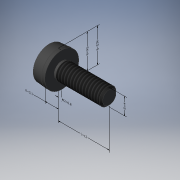
# Autodesk Inventor part: ART 48240 - DIN 6900-1 Z0 T M4x12.0 mm - A2
Saved by Autodesk Inventor 2019 (Build 230136000, 136)
## iProperties
Created: 2022-09-09
Part Number: ART 48240 - DIN 6900-1 Z0 T M4x12.0 mm - A2
Material: Generic
Catalog Web Link: www.cadenas.de
Description: DIN 6900-1 Z0 T stainless steel A2 plain-Torx SEMS screws with small flat washer
Vendor: ART
Document SubType Name: Modeling
Designer: psAdmin
Manufacturer: ART
Mass: 0.285727 g
Surface Area: 3.33062 cm^2
Volume: 0.285727 cm^3
Density: 1 g/cm^3
Appearance: PSOLRGB-192-192-192
Category: PARTsolutions
Company: ART
Title: A.R.T. 48240 - DIN 6900-1 Z0 T M4x12.0 mm - A2
Author: Cadenas PARTsolutions
Comments: Torx SEMS screws with small flat washer
PSOL_IDENT_0: {$CADENAS_DATA/23d-libs/art/mz/kombischrauben/din_6900_1_z1_z0_t/din_6900_1_z0_t_a2.prj},264 {VTYP=3
PSOL_IDENT_1: D},{NB=ART 48240 - DIN 6900-1 Z0 T M4x12.0 mm - A2},{LINA=A.R.T. 48240 - DIN 6900-1 Z0 T M4x12.0 mm
PSOL_IDENT_2: - A2},{NN=DIN 6900-1 Z0 T stainless steel A2 plain},{DATE=17.05.2021 04:49:58},{GEOMDATE=29.04.2021
PSOL_IDENT_3: 06:09:35},{VERSION=},{LINEID=260},{WBVAR=},{WBNUMERIC=}  {NB=ART 48240 - DIN 6900-1 Z0 T M4x12.0 mm
PSOL_IDENT_4: - A2},{LINA=A.R.T. 48240 - DIN 6900-1 Z0 T M4x12.0 mm - A2},{KT=X},{IDNR=},{NENN=M4x12.0 mm - A2},{A
PSOL_IDENT_5: RTNR=48240},{TYP=DIN 6900-1 Z0 T},{ZTN=7318 1595},{MT=Metall},{MAT=Edelstahl},{GUETE=A2},{OBERFLAECH
PSOL_IDENT_6: E=blank},{DINSCHRAUBE=DIN 7985 - Torx},{DINSCHEIBE=DIN 6902C - Unterlegscheibe ähnl. DIN 433 (Z0)},{
PSOL_IDENT_7: ISO=ISO 10644 S11-S},{D=4.0},{D3=3.141},{P=0.700},{L=12},{A=1.400},{B=10.6},{BX=22},{DK=8},{AD2=8.0}
PSOL_IDENT_8: ,{K=3.1},{H2=0.8},{ANTRIEB=Torx T20},{ANTRIEB1=Torx},{A1=3.950},{T=1.660},{DA=4.700},{R=0.200},{RF=8
PSOL_IDENT_9: .000},{V=2.000},{X=1.750},{DIN962FTHREAD=0},{VERS=1},{DIST=0.8},{CNSAVOID=0},{CNSNN=DIN 7985},{CNSOR
PSOL_IDENT_10: DER=DIN 7985 M4x12.0 mm - A2},{LINK1=www.artgmbh.com},{LWS=https://www.artgmbh.com/montagezubehoer-k
PSOL_IDENT_11: ombischrauben/kombischrauben/din-6900-1-z1-kombischrauben-torx-mit-unterlegscheibe/},{LINK2=https://
PSOL_IDENT_12: www.artgmbh.com/media/static/pdf/ART_ELEKTROMECHANIK_Gesamtkatalog.pdf},{LKS=https://www.artgmbh.com
PSOL_IDENT_13: /media/static/pdf/ART_ELEKTROMECHANIK_Gesamtkatalog.pdf}
NB: ART 48240 - DIN 6900-1 Z0 T M4x12.0 mm - A2
NN: DIN 6900-1 Z0 T stainless steel A2 plain
NT: Torx SEMS screws with small flat washer
NBSYN: ART $ARTNR. - $TYP. $NENN.
LINA: A.R.T. 48240 - DIN 6900-1 Z0 T M4x12.0 mm - A2
CATALOG: A.R.T. Elektromechanik
ROWDESC: M4x12.0 mm - A2
OFFICIAL_STANDARD_NUMBERS: DIN 6900
ARTNR: 48240
TYP: DIN 6900-1 Z0 T
ZTN: 7318 1595
MT: Metal
MAT: stainless steel
GUETE: A2
OBERFLAECHE: plain
DINSCHRAUBE: DIN 7985 - Torx
DINSCHEIBE: DIN 6902C - Flat washer similar to DIN 433 (Z0)
ISO: ISO 10644 S11-S
D: 4
P: 0.7
L: 12
DK: 8
AD2: 8
K: 3.1
H2: 0.8
ANTRIEB: Torx T20
LINK1: www.artgmbh.com
LINK2: https://www.artgmbh.com/media/static/pdf/ART_ELEKTROMECHANIK_Gesamtkatalog.pdf
SUPPLIER: ART
ARTICLENO: ART 48240 - DIN 6900-1 Z0 T M4x12.0 mm - A2
BOMINFO: A.R.T. 48240 - DIN 6900-1 Z0 T M4x12.0 mm - A2
CREATOR: CADENAS GmbH
Autodesk Inventor part; units mm, degrees
sketch "Skizze_3" plane through (0, 0, 0) normal (0, 0, 1) x (1, 0, 0)
  line L0 (12, 0) -> (-3.1, 0)
  line L1 (-3.1, 0) -> (-3.1, 4)
  line L2 (-3.1, 4) -> (0, 4)
  line L3 (0, 4) -> (0, 2)
  line L4 (0, 2) -> (11.5705, 2)
  line L5 (11.5705, 2) -> (12, 1.5705)
  line L6 (12, 1.5705) -> (12, 0)
  line L7 (12, 0) -> (-3.1, 0)
  constraints: 16 end point
revolve "Revolution1" add sketch "Skizze_3" angle 360 about axis through (12, 0, 0) along (1, 0, 0)
thread "Thread1" size "M4x0.7" class "6g" standard "ISO Metric profile" length 10.1705
sketch "Sketch_6" plane through (0, 0, 0) normal (0, 0, 1) x (1, 0, 0)
  line L0 (1.4, 0) -> (0, 0)
  line L1 (0, 2.6111) -> (0, 2.35)
  arc A0 (0, 2.35) -> (0.0908, 2.1825) centre (0.2, 2.35) ccw
  line L2 (0.0908, 2.1825) -> (0.7, 1.7853)
  line L3 (0.7, 1.7853) -> (1.4, 2)
  line L4 (1.4, 2) -> (1.4, 2.6111)
  line L5 (1.4, 2.6111) -> (0, 2.6111)
  constraints: 12 end point, 2 point on circle, 1 centre point
revolve "Revolution2" cut sketch "Sketch_6" angle 360 about axis through (1.4, 0, 0) along (1, 0, 0)
sketch "Sketch_2" plane through (0, 0, 0) normal (0, 0, 1) x (1, 0, 0)
  line L0 (0.7, 0) -> (-0.2, 0)
  line L1 (-0.2, 2.6111) -> (-0.2, 1.5705)
  line L2 (-0.2, 1.5705) -> (0.7, 1.5705)
  line L3 (0.7, 1.5705) -> (0.7, 1.7853)
  line L4 (0.7, 1.7853) -> (0.0908, 2.1825)
  arc A0 (0, 2.35) -> (0.0908, 2.1825) centre (0.2, 2.35) ccw
  line L5 (0, 2.35) -> (0, 2.6111)
  line L6 (0, 2.6111) -> (-0.2, 2.6111)
  constraints: 14 end point, 2 point on circle, 1 centre point
revolve "Revolution3" add sketch "Sketch_2" angle 360 about axis through (0.7, 0, 0) along (1, 0, 0)
sketch "Sketch_5" plane through (0, 0, 0) normal (0, 0, 1) x (1, 0, 0)
  line L0 (-3.1, 0) -> (-3.41, 0)
  line L1 (-3.41, 0) -> (-3.41, 4.4444)
  line L2 (-3.41, 4.4444) -> (0, 4.4444)
  line L3 (0, 4.4444) -> (0, 4)
  line L4 (0, 4) -> (-2.1326, 3.8134)
  arc A0 (-2.1326, 3.8134) -> (-3.1, 0) centre (4.9, 0) ccw
  line L5 (-3.1, 0) -> (-3.41, 0)
  constraints: 12 end point, 2 point on circle, 1 centre point
sketch "Sketch_1" plane through (0, 0, 0) normal (0, 0, 1) x (1, 0, 0)
  line L0 (-0.2997, 0) -> (-4.1, 0)
  line L1 (-4.1, 0) -> (-4.1, 1.975)
  line L2 (-4.1, 1.975) -> (-1.44, 1.975)
  line L3 (-1.44, 1.975) -> (-0.2997, 0)
  line L4 (-0.2997, 0) -> (-4.1, 0)
  constraints: 10 end point
revolve "Revolution4" cut sketch "Sketch_1" angle 360 about axis through (-0.2997, 0, 0) along (1, 0, 0)
sketch "Sketch_4" plane through (-3.1, 0, 0) normal (1, 0, 0) x (0, 0, -1)
  circle A0 centre (0, 0) radius 2.37
  arc A1 (-1.6394, -0.5027) -> (-1.2551, -1.1684) centre (-1.3683, -0.79) ccw
  arc A2 (-0.3843, -1.6711) -> (-1.2551, -1.1684) centre (-1.0569, -1.8307) ccw
  arc A3 (-0.3843, -1.6711) -> (0.3843, -1.6711) centre (0, -1.58) ccw
  arc A4 (1.2551, -1.1684) -> (0.3843, -1.6711) centre (1.0569, -1.8307) ccw
  arc A5 (1.2551, -1.1684) -> (1.6394, -0.5027) centre (1.3683, -0.79) ccw
  arc A6 (1.6394, 0.5027) -> (1.6394, -0.5027) centre (2.1139, 0) ccw
  arc A7 (1.6394, 0.5027) -> (1.2551, 1.1684) centre (1.3683, 0.79) ccw
  arc A8 (0.3843, 1.6711) -> (1.2551, 1.1684) centre (1.0569, 1.8307) ccw
  arc A9 (0.3843, 1.6711) -> (-0.3843, 1.6711) centre (0, 1.58) ccw
  arc A10 (-1.2551, 1.1684) -> (-0.3843, 1.6711) centre (-1.0569, 1.8307) ccw
  arc A11 (-1.2551, 1.1684) -> (-1.6394, 0.5027) centre (-1.3683, 0.79) ccw
  arc A12 (-1.6394, -0.5027) -> (-1.6394, 0.5027) centre (-2.1139, 0) ccw
  constraints: 24 point on circle, 13 centre point
extrude "Extrusion1" add sketch "Sketch_4" along normal blind 2.49
sketch "Sketch_8" plane through (0, 0, 0) normal (0, 0, 1) x (1, 0, 0)
  line L0 (-1.9597, 0) -> (-4.76, 0)
  line L1 (-4.76, 0) -> (-4.76, 1.975)
  line L2 (-4.76, 1.975) -> (-3.1, 1.975)
  line L3 (-3.1, 1.975) -> (-1.9597, 0)
  line L4 (-1.9597, 0) -> (-4.76, 0)
  constraints: 10 end point
revolve "Revolution5" cut sketch "Sketch_8" angle 360 about axis through (-1.9597, 0, 0) along (1, 0, 0)
revolve "Revolution6" cut sketch "Sketch_5" angle 360 about axis through (-3.1, 0, 0) along (1, 0, 0)
sketch "Sketch_9" plane through (0, 0, 0) normal (0, 0, 1) x (1, 0, 0)
  line L0 (0.8, 0) -> (0, 0)
  line L1 (0, 0) -> (0, 4)
  line L2 (0, 4) -> (0.8, 4)
  line L3 (0.8, 4) -> (0.8, 0)
  line L4 (0.8, 0) -> (0, 0)
  constraints: 10 end point
revolve "Revolution7" add sketch "Sketch_9" angle 360 about axis through (0.8, 0, 0) along (1, 0, 0)
ref_plane "IP1_XY" through (0, 0, 0) normal (1, 0, 0) x (0, 0, -1)
ref_plane "IP1_YZ" through (0, 0, 0) normal (0, 0, -1) x (0, 1, 0)
ref_plane "IP1_ZX" through (0, 0, 0) normal (0, 1, 0) x (1, 0, 0)
ref_plane "IP2_XY" through (-3.1, 0, 0) normal (1, 0, 0) x (0, 0, -1)
ref_plane "IP2_YZ" through (-3.1, 0, 0) normal (0, 0, -1) x (0, 1, 0)
ref_plane "IP2_ZX" through (-3.1, 0, 0) normal (0, 1, 0) x (1, 0, 0)
ref_plane "IP3_XY" through (12, 0, 0) normal (1, 0, 0) x (0, 0, -1)
ref_plane "IP3_YZ" through (12, 0, 0) normal (0, 0, -1) x (0, 1, 0)
ref_plane "IP3_ZX" through (12, 0, 0) normal (0, 1, 0) x (1, 0, 0)
body "Solid1"
